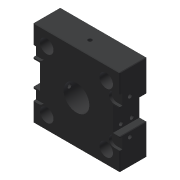
# Autodesk Inventor part: bottomplate2
Saved by Autodesk Inventor 2022 Beta2 (Build 260130000, 130) ContinuousBuild 0
## iProperties
Shininess: 64.0
Length Units: 11272
Angle Units: 11279
Time Units: 11290
Mass Units: 11286
Length Display Precision: 3
Angle Display Precision: 2
Compacted: True
Part Number: bottomplate2
Document SubType Name: Modeling
Created: 2003-04-03
Designer: Sudhir John
Density: 1 g/cm^3
Material: Generic
Appearance: Generic
Density: 0.0
Volumn: 0.0
Area: 0.0
PropertySet Name: Model Information
Control State: 0
Master: False
Checked Out: False
Author: Sudhir John
Autodesk Inventor part; units mm, degrees
sketch "Sketch1" plane through (0, 0, 0) normal (0, 0, 1) x (1, 0, 0)
  line L0 (-14.9871, -174.324) -> (188.2129, -174.324)
  line L1 (188.2129, -174.324) -> (188.2129, 28.876)
  line L2 (188.2129, 28.876) -> (-14.9871, 28.876)
  line L3 (-14.9871, 28.876) -> (-14.9871, -174.324)
  dimension "d0" = 203.2
  dimension "d1" = 203.2
  constraints: 8 end point, 2 parallel, 1 horizontal, 1 perpendicular
  measures "d0" distance of L1.end L2.end
  measures "d1" distance of L2.end L0.start
extrude "Extrusion1" add sketch "Sketch1" along normal blind 63.5
ref_plane "Work Plane1" through (-14.9871, -72.724, 0) normal (0, 1, 0) x (1, 0, 0)
ref_plane "Work Plane2" through (86.6129, -174.324, 0) normal (1, 0, 0) x (0, 0, -1)
sketch "Sketch2" plane through (0, 0, 63.5) normal (0, 0, 1) x (1, 0, 0)
  line L0 (-14.9871, -174.324) -> (-14.9871, 28.876) projected
  line L1 (-35.3071, -72.724) -> (249.1729, -72.724) projected
  line L2 (-14.9871, -44.149) -> (1.0149, -44.149)
  line L3 (1.0149, -44.149) -> (1.0149, -101.299)
  line L4 (1.0149, -101.299) -> (-14.9871, -101.299)
  line L5 (-14.9871, -101.299) -> (-14.9871, -44.149)
  dimension "d4" = 57.15
  dimension "d5" = 28.575
  dimension "d6" = 16.002
  constraints: 8 end point, 2 parallel, 1 horizontal, 1 perpendicular, 1 point on line
  measures "d4" distance of L2.end L3.end
  measures "d5" distance between parallel lines of L1 L4
  measures "d6" distance of L3.end L4.end
extrude "Extrusion2" cut sketch "Sketch2" against normal through all
mirror "Mirror1" about plane through (86.6129, -174.324, 0) normal (1, 0, 0) of "Extrusion2"
sketch "Sketch3" plane through (-14.9871, -72.724, 0) normal (0, 1, 0) x (1, 0, 0)
  line L0 (101.6, 6.35) -> (101.6, -82.55) projected
  line L1 (101.6, -63.5) -> (131.7625, -63.5)
  line L2 (131.7625, -63.5) -> (131.7625, -54.4576)
  line L3 (131.7625, -54.4576) -> (133.63, -53.1779)
  line L4 (133.63, -53.1779) -> (133.63, -10.4297)
  line L5 (133.63, -10.4297) -> (134.9502, -9.525)
  line L6 (134.9502, -9.525) -> (134.9502, 0)
  line L7 (134.9502, 0) -> (101.6, 0)
  line L8 (203.2, 0) -> (0, 0) projected
  line L9 (0, -63.5) -> (203.2, -63.5) projected
  dimension "d9" = 30.1625
  dimension "d10" = 9.0424
  dimension "d11" = 42.7482
  dimension "d12" = 9.525
  dimension "d13" = 33.3502
  constraints: 14 end point, 3 parallel, 3 perpendicular, 2 collinear, 2 point on line
  measures "d9" distance of L1.start L1.end
  measures "d10" distance of L1.end L2.end
  measures "d11" distance of L3.end L4.end
  measures "d12" distance of L5.end L6.end
  measures "d13" distance between parallel lines of L0 L6
revolve "Revolution1" cut sketch "Sketch3" angle 360 about axis through (86.6129, -72.724, 0) along (0, 0, 1)
sketch "Sketch4" plane through (0, 0, 0) normal (0, 0, -1) x (-1, 0, 0)
  line L0 (-188.2129, 28.876) -> (14.9871, 28.876) projected
  line L1 (-188.2129, -44.149) -> (-188.2129, 28.876) projected
  line L2 (-86.6129, -194.644) -> (-86.6129, 89.836) projected
  line L3 (-249.1729, -72.724) -> (35.3071, -72.724) projected
  point P0 (-156.4629, -2.874)
  point P1 (-16.7629, -2.874)
  point P2 (-156.4629, -142.574)
  point P3 (-16.7629, -142.574)
  dimension "d15" = 31.75
  dimension "d16" = 31.75
  constraints: 3 symmetric about line
  measures "d15" distance from line of L0 point (-156.463, -2.874)
  measures "d16" distance from line of L1 point (-156.463, -2.874)
hole "Hole1" at (156.4629, -2.874, 0) at (16.7629, -2.874, 0) at (156.4629, -142.574, 0) at (16.7629, -142.574, 0) direction (0, 0, 1) diameter 31.75 end through all counterbore diameter 37.084 counterbore depth 5.08
sketch "Sketch5" plane through (0, 0, 63.5) normal (0, 0, 1) x (1, 0, 0)
  line L0 (-14.9871, -174.324) -> (-14.9871, -101.299) projected
  line L1 (188.2129, -174.324) -> (-14.9871, -174.324) projected
  line L2 (-14.9871, -104.474) -> (-2.2871, -104.474)
  line L3 (-2.2871, -129.874) -> (-14.9871, -129.874)
  line L4 (-14.9871, -129.874) -> (-14.9871, -104.474)
  arc A0 (-2.2871, -129.874) -> (-2.2871, -104.474) centre (-2.2871, -117.174) ccw
  dimension "d24" = 44.45
  dimension "d26" = 12.7
  constraints: 6 end point, 2 point on circle, 1 centre point, 1 horizontal, 1 parallel, 1 point on line
  measures "d24" distance between parallel lines of L1 L3
  measures "d26" distance of L3.start L3.end
extrude "Extrusion3" cut sketch "Sketch5" against normal blind 6.35
mirror "Mirror2" about plane through (86.6129, -174.324, 0) normal (1, 0, 0) of "Extrusion3"
mirror "Mirror3" about plane through (-14.9871, -72.724, 0) normal (0, 1, 0) of "Extrusion3", "Mirror2"
sketch "Sketch6" plane through (-14.9871, -174.324, 0) normal (0, -1, 0) x (1, 0, 0)
  line L0 (203.2, 63.5) -> (0, 63.5) projected
  line L1 (101.6, 82.55) -> (101.6, -6.35) projected
  point P0 (142.24, 48.26)
  point P1 (60.96, 48.26)
  dimension "d29" = 15.24
  dimension "d30" = 40.64
  constraints: 1 symmetric about line
  measures "d29" distance from line of L0 point (142.24, 48.26)
  measures "d30" distance from line of L1 point (142.24, 48.26)
hole "Hole2" at (127.2529, -174.324, 48.26) at (45.9729, -174.324, 48.26) direction (0, 1, 0) diameter 9.144 depth 101.6 tip angle 118 counterbore diameter 25.4 counterbore depth 25.4 thread size "7/16-14 UNC" class "1B" standard "ANSI Unified Screw Threads"
sketch "Sketch7" plane through (-14.9871, -174.324, 0) normal (0, -1, 0) x (1, 0, 0)
  line L0 (0, 0) -> (203.2, 0) projected
  point P0 (60.96, 23.368)
  point P1 (142.24, 23.368)
  dimension "d38" = 23.368
  measures "d38" distance from line of L0 point (60.96, 23.368)
hole "Hole3" at (45.9729, -174.324, 23.368) at (127.2529, -174.324, 23.368) direction (0, 1, 0) diameter 9.144 depth 101.6 tip angle 118 counterbore diameter 19.05 counterbore depth 17.4498 thread size "7/16-14 UNC" class "1B" standard "ANSI Unified Screw Threads"
ref_plane "Work Plane3" through (0, 0, 31.75) normal (0, 0, 1) x (1, 0, 0)
sketch "Sketch8" plane through (172.2109, -101.6229, 6.5724) normal (1, 0, 0) x (0, 0, -1)
  line L0 (-25.4, -93.345) -> (-25.4, 191.135)
  line L1 (-66.04, 28.575) -> (5.08, 28.575)
  point P0 (-38.1, 47.625)
  point P1 (-12.7, 47.625)
  point P2 (-38.1, 9.525)
  point P3 (-12.7, 9.525)
  dimension "d48" = 12.7
  dimension "d47" = 19.05
  constraints: 4 end point, 3 symmetric about line
  measures "d48" distance from line of L0 point (-38.1, 47.625)
  measures "d47" distance from line of L1 point (-38.1, 47.625)
hole "Hole4" at (172.2109, -53.9979, 44.6724) at (172.2109, -53.9979, 19.2724) at (172.2109, -92.0979, 44.6724) at (172.2109, -92.0979, 19.2724) direction (-1, 0, 0) diameter 9.144 depth 18.8468 tip angle 118
mirror "Mirror4" about plane through (86.6129, -174.324, 0) normal (1, 0, 0) of "Hole4"
sketch "Sketch9" plane through (188.2129, -173.8086, 63.0266) normal (1, 0, 0) x (0, 0, -1)
  line L0 (0, 73.025) -> (0, 0)
  line L1 (-2.794, 101.6) -> (68.326, 101.6)
  point P0 (23.622, 60.325)
  point P1 (23.622, 142.875)
  dimension "d57" = 41.275
  dimension "d56" = 23.622
  constraints: 4 end point, 1 symmetric about line
  measures "d57" distance from line of L1 point (23.622, 60.325)
  measures "d56" distance from line of L0 point (23.622, 60.325)
hole "Hole5" at (188.2129, -113.4836, 39.4046) at (188.2129, -30.9336, 39.4046) direction (-1, 0, 0) diameter 9.144 depth 32.4612 tip angle 118
mirror "Mirror6" about plane through (86.6129, -174.324, 0) normal (1, 0, 0) of "Hole5"
sketch "Sketch10" plane through (-14.9871, -174.324, 0) normal (0, -1, 0) x (1, 0, 0)
  line L0 (101.6, 82.55) -> (101.6, -6.35) projected
  line L1 (-20.32, 31.75) -> (264.16, 31.75) projected
  point P0 (101.6, 31.75)
  point P1 (142.0313, -66.6979)
  constraints: 2 point on line
hole "Hole6" at (86.6129, -174.324, 31.75) at (127.0442, -174.324, -66.6979) direction (0, 1, 0) diameter 9.144 depth 26.1112 tip angle 118 thread size "7/16-14 UNC" class "1B" standard "ANSI Unified Screw Threads"
mirror "Mirror5" about plane through (-14.9871, -72.724, 0) normal (0, 1, 0) of "Hole6"
sketch "Sketch11" plane through (0, 0, 0) normal (0, 0, -1) x (-1, 0, 0)
  line L0 (-188.2129, -174.324) -> (-188.2129, -101.299) projected
  line L1 (14.9871, -174.324) -> (-188.2129, -174.324) projected
  line L2 (-86.6129, -194.644) -> (-86.6129, 89.836) projected
  line L3 (-249.1729, -72.724) -> (35.3071, -72.724) projected
  point P0 (-86.6129, -123.524)
  point P1 (-150.1129, -110.824)
  point P2 (-23.1129, -110.824)
  point P3 (-150.1129, -34.624)
  point P4 (-23.1129, -34.624)
  point P5 (-86.6129, -21.924)
  dimension "d71" = 50.8
  dimension "d72" = 38.1
  dimension "d73" = 63.5
  constraints: 4 symmetric about line, 1 point on line
  measures "d71" distance from line of L1 point (-86.613, -123.524)
  measures "d72" distance from line of L0 point (-150.113, -110.824)
  measures "d73" distance from line of L1 point (-150.113, -110.824)
hole "Hole7" at (86.6129, -123.524, 0) at (150.1129, -110.824, 0) at (23.1129, -110.824, 0) at (150.1129, -34.624, 0) at (23.1129, -34.624, 0) at (86.6129, -21.924, 0) direction (0, 0, 1) diameter 9.144 depth 32.4612 tip angle 118 thread size "7/16-14 UNC" class "1B" standard "ANSI Unified Screw Threads"
sketch "Sketch12" plane through (1.0149, -101.299, 63.5) normal (-1, 0, 0) x (0, 0, 1)
  line L0 (0, 57.15) -> (0, 0) projected
  line L1 (-69.85, 28.575) -> (19.05, 28.575) projected
  point P0 (-15.4686, 28.575)
  dimension "d81" = 15.4686
  constraints: 1 point on line
  measures "d81" distance from line of L0 point (-15.469, 28.575)
hole "Hole8" at (1.0149, -72.724, 48.0314) direction (1, 0, 0) diameter 9.144 depth 127 tip angle 118 thread size "7/16-14 UNC" class "1B" standard "ANSI Unified Screw Threads"
sketch "Sketch13" plane through (1.0149, -101.299, 63.5) normal (-1, 0, 0) x (0, 0, 1)
  circle A0 centre (-15.4686, 28.575) radius 4.572 projected
  line L0 (-69.85, 28.575) -> (19.05, 28.575) projected
  point P0 (-40.132, 28.575)
  dimension "d90" = 24.6634
  constraints: 1 point on line
  measures "d90" distance of A0.centre point (-40.132, 28.575)
hole "Hole9" at (1.0149, -72.724, 23.368) direction (1, 0, 0) diameter 9.144 depth 127 tip angle 118 thread size "7/16-14 UNC" class "1B" standard "ANSI Unified Screw Threads"
chamfer "Chamfer1" distance 1.27 angle 45 26 edges at (86.6129, 28.876, 63.5) (-14.9871, 28.876, 31.75) (86.6129, 28.876, 0) (188.2129, 28.876, 31.75) (-14.9871, 6.651, 63.5) (-14.9871, -42.5615, 63.5) (-14.9871, -102.8865, 63.5) (-14.9871, -152.099, 63.5) (86.6129, -174.324, 63.5) (188.2129, -152.099, 63.5) (188.2129, -102.8865, 63.5) (188.2129, -42.5615, 63.5) (188.2129, 6.651, 63.5) (188.2129, -7.6365, 0) (188.2129, -137.8115, 0) (188.2129, -174.324, 31.75) (188.2129, -101.299, 31.75) (172.2109, -72.724, 0) (180.2119, -44.149, 0) (180.2119, -101.299, 0) (86.6129, -174.324, 0) (-14.9871, -137.8115, 0) (-6.9861, -101.299, 0) (1.0149, -72.724, 0) (-6.9861, -44.149, 0) (-14.9871, -7.6365, 0)
body "Solid1"
